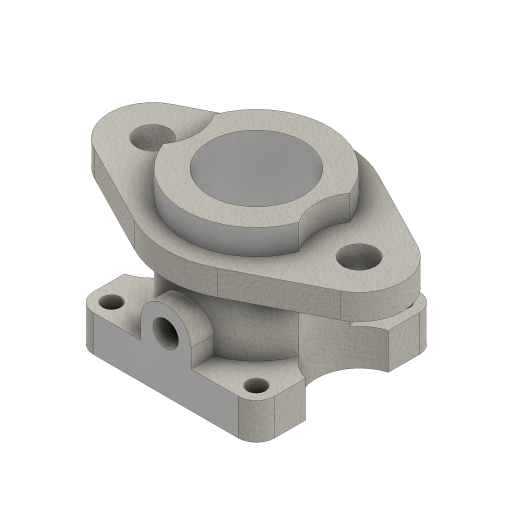
# Autodesk Inventor part: Part025. Connection body
Saved by Autodesk Inventor 2023.2 (Build 272271030, 271C)
## iProperties
Created: 2023-10-06
Part Number: Part025. Connection body
Material: Steel, Carbon
Document SubType Name: Modeling
Designer: User
Mass: 373.024 g
Surface Area: 175.038 cm^2
Volume: 47.519 cm^3
Density: 7.85 g/cm^3
Appearance: Steel - Cast
Author: User
Autodesk Inventor part; units mm, degrees
note: some values were not read from the file. Chosen so that the rebuilt part matches the saved one: direction of "Hole2".
ref_plane "YZ Plane" through (0, 0, 0) normal (1, 0, 0) x (0, 1, 0)
ref_plane "XZ Plane" through (0, 0, 0) normal (0, 1, 0) x (-1, 0, 0)
sketch "Sketch1" plane through (0, 0, 0) normal (0, 1, 0) x (-1, 0, 0)
  line L0 (25, 25) -> (-25, 25)
  line L1 (-25, 25) -> (-25, -25)
  line L2 (-25, -25) -> (25, -25)
  line L3 (25, -25) -> (25, 25)
  line L4 (25, 25) -> (-25, -25) construction
  line L5 (-25, 25) -> (25, -25) construction
  point P0 (0, 0)
  dimension "d0" = 50
  dimension "d1" = 50
  constraints: 12 end point, 2 midpoint, 2 parallel, 1 horizontal, 1 perpendicular
  measures "d0" distance of L2.end L1.end
  measures "d1" distance of L1.end L0.end
extrude "Extrusion1" add sketch "Sketch1" along normal blind 10
fillet "Fillet1" radius 5 4 edges at (-25, 5, -25) (-25, 5, 25) (25, 5, -25) (25, 5, 25)
sketch "Sketch2" plane through (0, 10, 0) normal (0, 1, 0) x (1, 0, 0)
  circle A0 centre (0, 0) radius 20
  dimension "d5" = 40
  constraints: 1 centre point, 1 coincident
  measures "d5" diameter of A0
extrude "Extrusion2" add sketch "Sketch2" along normal blind 32
sketch "Sketch4" plane through (0, 0, 0) normal (0, -1, 0) x (1, 0, 0)
  circle A0 centre (-28.5, 0) radius 12
  line L0 (0, -36.4497) -> (0, 36.4497) projected
  circle A1 centre (28.5, 0) radius 12
  point P0 (0, 0)
  dimension "d14" = 12
  dimension "d15" = 57
  constraints: 2 centre point, 1 horizontal alignment, 1 symmetric about line, 1 other
  measures "d14" radius of A0
  measures "d15" distance of A1.centre A0.centre
extrude "Extrusion4" cut sketch "Sketch4" against normal through all
ref_plane "Work Plane1" through (0, 28, 0) normal (0, -1, 0) x (1, 0, 0)
sketch "Sketch3" plane through (0, 28, 0) normal (0, -1, 0) x (1, 0, 0)
  line L0 (-34.0605, -10.6894) -> (-11.3607, -22.2696)
  arc A0 (-11.3607, -22.2696) -> (11.4466, -22.2255) centre (0, 0) ccw
  line L1 (11.4466, -22.2255) -> (33.887, -10.6683)
  line L2 (33.887, -10.6683) -> (33.887, -10.6683)
  arc A1 (33.887, -10.6683) -> (33.887, 10.6683) centre (28.3926, 0) ccw
  line L3 (33.887, 10.6683) -> (11.4466, 22.2255)
  arc A2 (11.4466, 22.2255) -> (-11.3607, 22.2696) centre (0, 0) ccw
  arc A3 (-34.0605, 10.6894) -> (-34.0605, -10.6894) centre (-28.6074, 0) ccw
  line L4 (-11.3607, 22.2696) -> (-34.0605, 10.6894)
  dimension "d9" = 25
  dimension "d10" = 12
  dimension "d11" = 57
  constraints: 10 end point, 8 point on circle, 8 tangent, 4 centre point, 2 coincident, 2 equal radius, 2 horizontal alignment
  measures "d9" radius of A0
  measures "d10" radius of A1
  measures "d11" distance of A1.centre A3.centre
extrude "Extrusion3" add sketch "Sketch3" against normal blind 7
sketch "Sketch5" plane through (0, 42, 0) normal (0, 1, 0) x (1, 0, 0)
  arc A0 (18.7412, 6.9833) -> (-18.7412, 6.9833) centre (0, 0) ccw projected
  constraints: 1 coincident
hole "Hole1" at (0, 42, 0) direction (0, -1, 0) diameter 26 end through all
sketch "Sketch6" plane through (-20, 0, 25) normal (0, 0, 1) x (1, 0, 0)
  line L0 (0, 10) -> (40, 10) projected
  line L1 (0, 0) -> (40, 0) projected
  line L2 (1.2588, 10) -> (38.7412, 10) projected
  line L3 (13, 10) -> (13, 15)
  arc A0 (27, 15) -> (13, 15) centre (20, 15) ccw
  line L4 (27, 15) -> (27, 10)
  point P0 (20, 0)
  point P1 (20, 0)
  point P2 (20, 0)
  dimension "d25" = 7
  dimension "d26" = 15
  constraints: 4 end point, 2 midpoint, 2 perpendicular, 2 point on circle, 2 point on line, 2 tangent, 1 centre point, 1 vertical alignment
  measures "d25" radius of A0
  measures "d26" distance of point (20, 0) A0.centre
extrude "Extrusion5" add sketch "Sketch6" against normal up to surface
sketch "Sketch7" plane through (-20, 0, 25) normal (0, 0, 1) x (1, 0, 0)
  arc A0 (27, 15) -> (13, 15) centre (20, 15) ccw projected
  point P0 (20, 0)
  constraints: 1 coincident
hole "Hole2" at (0, 15, 25) direction (0, 0, -1) diameter 7 end up to surface
sketch "Sketch8" plane through (0, 10, 0) normal (0, 1, 0) x (1, 0, 0)
  arc A0 (-25, -20) -> (-20, -25) centre (-20, -20) ccw projected
  arc A1 (25, 11.4782) -> (18.7412, 6.9833) centre (28.5, 0) ccw projected
  line L0 (25, 11.4782) -> (25, 20) projected
  arc A2 (25, 20) -> (20, 25) centre (20, 20) ccw projected
  line L1 (20, 25) -> (-20, 25) projected
  arc A3 (-20, 25) -> (-25, 20) centre (-20, 20) ccw projected
  line L2 (-25, 20) -> (-25, 11.4782) projected
  arc A4 (-18.7412, 6.9833) -> (-25, 11.4782) centre (-28.5, 0) ccw projected
  arc A5 (18.7412, 6.9833) -> (-18.7412, 6.9833) centre (0, 0) ccw projected
  line L3 (7, -18.735) -> (7, -25) projected
  line L4 (7, -25) -> (20, -25) projected
  arc A6 (20, -25) -> (25, -20) centre (20, -20) ccw projected
  line L5 (25, -20) -> (25, -11.4782) projected
  arc A7 (18.7412, -6.9833) -> (25, -11.4782) centre (28.5, 0) ccw projected
  arc A8 (7, -18.735) -> (18.7412, -6.9833) centre (0, 0) ccw projected
hole "Hole3" at (-20, 10, 20) at (20, 10, 20) at (-20, 10, -20) at (20, 10, -20) direction (0, -1, 0) diameter 5 end through all
sketch "Sketch9" plane through (0, 35, 0) normal (0, 1, 0) x (1, 0, 0)
  arc A0 (-34.0605, 10.6894) -> (-34.0605, -10.6894) centre (-28.6074, 0) ccw projected
  arc A1 (33.887, -10.6683) -> (33.887, 10.6683) centre (28.3926, 0) ccw projected
  point P0 (0, 0)
  point P1 (-28.6074, 0)
  constraints: 2 coincident
hole "Hole4" at (-28.6074, 35, 0) at (28.3926, 35, 0) direction (0, -1, 0) diameter 9 end through all
body "Solid1"
